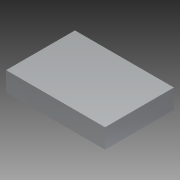
# Autodesk Inventor part: boundingbox
Saved by Autodesk Inventor 2013 SP2 (Build 170200200, 200)
## iProperties
Created: 2018-09-21
Part Number: boundingbox
Material: Generic
Document SubType Name: Modeling
Designer: alex
Density: 1 g/cm^3
Author: alex
Autodesk Inventor part; units mm, degrees
ref_plane "YZ Plane" through (0, 0, 0) normal (1, 0, 0) x (0, 1, 0)
ref_plane "XZ Plane" through (0, 0, 0) normal (0, 1, 0) x (-1, 0, 0)
ref_plane "XY Plane" through (0, 0, 0) normal (0, 0, 1) x (1, 0, 0)
sketch "Sketch1" plane through (0, 0, 0) normal (0, 0, 1) x (1, 0, 0)
  line L0 (-230, -160) -> (230, -160)
  line L1 (230, -160) -> (230, 160)
  line L2 (230, 160) -> (-230, 160)
  line L3 (-230, 160) -> (-230, -160)
  line L4 (-230, -160) -> (230, 160) construction
  line L5 (230, -160) -> (-230, 160) construction
  point P0 (0, 0)
  dimension "d0" = 460
  dimension "d1" = 320
  constraints: 12 end point, 2 midpoint, 2 parallel, 1 horizontal, 1 perpendicular
  measures "d0" distance of L2.end L1.end
  measures "d1" distance of L1.end L0.end
extrude "Extrusion1" add sketch "Sketch1" along normal blind 90
body "Solid1"
